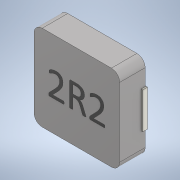
# Autodesk Inventor part: L_52x54x18mm
Saved by Autodesk Inventor 2020.3 (Build 243373000, 373)
## iProperties
Created: 2020-07-25
Part Number: L_52x54x18mm
Material: Generic
Document SubType Name: Modeling
Designer: franc
Density: 1 g/cm^3
Appearance: Default
Author: franc
Autodesk Inventor part; units mm, degrees
ref_plane "YZ Plane" through (0, 0, 0) normal (1, 0, 0) x (0, 1, 0)
ref_plane "XZ Plane" through (0, 0, 0) normal (0, 1, 0) x (-1, 0, 0)
ref_plane "XY Plane" through (0, 0, 0) normal (0, 0, 1) x (1, 0, 0)
sketch "Sketch1" plane through (0, 0, 0) normal (0, 0, 1) x (1, 0, 0)
  line L0 (-2.6, 2.6) -> (2.6, 2.6)
  line L1 (2.6, 2.6) -> (2.6, -2.6)
  line L2 (2.6, -2.6) -> (-2.6, -2.6)
  line L3 (-2.6, -2.6) -> (-2.6, 2.6)
  line L4 (-2.6, 2.6) -> (2.6, -2.6) construction
  line L5 (2.6, 2.6) -> (-2.6, -2.6) construction
  point P0 (0, 0)
  dimension "d0" = 5.2
  dimension "d1" = 5.2
  constraints: 12 end point, 2 midpoint, 2 parallel, 1 horizontal, 1 perpendicular
  measures "d0" distance of L0.start L0.end
  measures "d1" distance of L0.end L1.end
extrude "Extrusion1" add sketch "Sketch1" along normal blind 1.55
sketch "Sketch2" plane through (0, 0, 0) normal (0, 0, -1) x (-1, 0, 0)
  line L0 (-1.5, -1.1) -> (-2.7, -1.1)
  line L1 (-2.7, -1.1) -> (-2.7, 1.1)
  line L2 (-2.7, 1.1) -> (-1.5, 1.1)
  line L3 (-1.5, 1.1) -> (-1.5, -1.1)
  line L4 (-1.5, -1.1) -> (-2.7, 1.1) construction
  line L5 (-2.7, -1.1) -> (-1.5, 1.1) construction
  line L6 (-2.6, -2.6) -> (-2.6, 2.6) construction
  line L7 (-2.6, 0) -> (2.6, 0) construction
  line L8 (2.6, 2.6) -> (2.6, -2.6) construction
  line L9 (-2.6, 2.6) -> (2.6, 2.6) construction
  line L10 (0, 2.6) -> (0, 0) construction
  line L11 (1.5, -1.1) -> (2.7, -1.1)
  line L12 (2.7, -1.1) -> (2.7, 1.1)
  line L13 (2.7, 1.1) -> (1.5, 1.1)
  line L14 (1.5, 1.1) -> (1.5, -1.1)
  point P0 (-2.1, 0)
  point P1 (-2.1, 0)
  point P2 (2.1, 0)
  point P3 (2.1, 0)
  dimension "d4" = 1.2
  dimension "d5" = 0.1
  dimension "d6" = 2.2
  dimension "d7" = 5.4
  constraints: 24 end point, 6 midpoint, 6 symmetric about line, 2 parallel, 1 horizontal, 1 perpendicular, 1 point on line, 1 vertical
  measures "d4" distance of L0.start L0.end
  measures "d5" distance between parallel lines of L6 L1
  measures "d6" distance of L0.end L1.end
  measures "d7" distance between parallel lines of L12 L1
extrude "Extrusion2" add sketch "Sketch2" along normal blind 0.05 and the other way blind 0.25
fillet "Fillet1" radius 0.5 4 edges at (2.6, 2.6, 0.775) (-2.6, 2.6, 0.775) (2.6, -2.6, 0.775) (-2.6, -2.6, 0.775)
sketch "Sketch3" plane through (0, 0, 1.55) normal (0, 0, 1) x (1, 0, 0)
  line L0 (-2.5, 1.25) -> (2.5, 1.25) construction
  line L1 (2.5, 1.25) -> (2.5, -1.25) construction
  line L2 (2.5, -1.25) -> (-2.5, -1.25) construction
  line L3 (-2.5, -1.25) -> (-2.5, 1.25) construction
  line L4 (2.1, 2.6) -> (-2.1, 2.6) construction
  line L5 (0, 2.6) -> (0, -2.6) construction
  line L6 (-2.1, -2.6) -> (2.1, -2.6) construction
  line L7 (-2.6, 1.1) -> (-2.6, -1.1) construction
  line L8 (-2.6, 0) -> (2.6, 0) construction
  line L9 (2.6, -1.1) -> (2.6, 1.1) construction
  spline S0 degree 2 poles (-0.7725, -0.6683) (-0.7725, -0.6894) (-0.7782, -0.7218) (-0.788, -0.7444) (-0.8063, -0.7542) (-0.8162, -0.7542) knots 0 0 0 1 2 3 4 4 4
  line L10 (-0.8162, -0.7542) -> (-1.6415, -0.7542)
  spline S1 degree 2 poles (-1.6415, -0.7542) (-1.6585, -0.7542) (-1.6824, -0.7458) (-1.6993, -0.7275) (-1.7077, -0.6923) (-1.7077, -0.6669) knots 0 0 0 1 2 3 4 4 4
  spline S2 degree 2 poles (-1.7077, -0.6669) (-1.7077, -0.6444) (-1.7035, -0.6092) (-1.6923, -0.5824) (-1.6739, -0.557) (-1.6599, -0.5415) knots 0 0 0 1 2 3 4 4 4
  line L11 (-1.6599, -0.5415) -> (-1.3613, -0.2345)
  spline S3 degree 2 poles (-1.3613, -0.2345) (-1.257, -0.1289) (-1.1317, 0.0401) (-1.0641, 0.1782) (-1.043, 0.2908) (-1.043, 0.3415) knots 0 0 0 1 2 3 4 4 4
  spline S4 degree 2 poles (-1.043, 0.3415) (-1.043, 0.3908) (-1.0768, 0.4796) (-1.1401, 0.5458) (-1.2345, 0.5852) (-1.2965, 0.5852) knots 0 0 0 1 2 3 4 4 4
  spline S5 degree 2 poles (-1.2965, 0.5852) (-1.3697, 0.5852) (-1.4852, 0.5458) (-1.5725, 0.5007) (-1.6303, 0.4613) (-1.6444, 0.4613) knots 0 0 0 1 2 3 4 4 4
  spline S6 degree 2 poles (-1.6444, 0.4613) (-1.6528, 0.4613) (-1.6669, 0.4711) (-1.6754, 0.4908) (-1.6796, 0.5261) (-1.6796, 0.55) knots 0 0 0 1 2 3 4 4 4
  spline S7 degree 2 poles (-1.6796, 0.55) (-1.6796, 0.5669) (-1.6768, 0.5923) (-1.6711, 0.612) (-1.6627, 0.6275) (-1.6345, 0.6514) (-1.5669, 0.6937) (-1.4641, 0.7331) (-1.3401, 0.7613) (-1.2725, 0.7613) knots 0 0 0 1 2 3 4 5 6 7 8 8 8
  spline S8 degree 2 poles (-1.2725, 0.7613) (-1.1641, 0.7613) (-1.0007, 0.7007) (-0.8937, 0.5937) (-0.8401, 0.4528) (-0.8401, 0.3739) knots 0 0 0 1 2 3 4 4 4
  spline S9 degree 2 poles (-0.8401, 0.3739) (-0.8401, 0.3021) (-0.8655, 0.1599) (-0.9472, -0.0049) (-1.1021, -0.2063) (-1.2317, -0.3387) knots 0 0 0 1 2 3 4 4 4
  line L12 (-1.2317, -0.3387) -> (-1.4683, -0.5852)
  line L13 (-1.4683, -0.5852) -> (-0.8176, -0.5852)
  spline S10 degree 2 poles (-0.8176, -0.5852) (-0.8077, -0.5852) (-0.7908, -0.5951) (-0.7782, -0.6162) (-0.7725, -0.6472) (-0.7725, -0.6683) knots 0 0 0 1 2 3 4 4 4
  spline S11 degree 2 poles (0.5528, -0.7246) (0.5528, -0.7331) (0.5458, -0.7472) (0.5232, -0.757) (0.481, -0.7613) (0.4472, -0.7613) knots 0 0 0 1 2 3 4 4 4
  spline S12 degree 2 poles (0.4472, -0.7613) (0.4162, -0.7613) (0.3782, -0.757) (0.3556, -0.7458) (0.343, -0.7275) (0.3387, -0.7134) knots 0 0 0 1 2 3 4 4 4
  line L14 (0.3387, -0.7134) -> (0.2007, -0.3627)
  spline S13 degree 2 poles (0.2007, -0.3627) (0.1768, -0.3021) (0.1246, -0.2021) (0.0528, -0.1303) (-0.043, -0.0894) (-0.112, -0.0894) knots 0 0 0 1 2 3 4 4 4
  line L15 (-0.112, -0.0894) -> (-0.2444, -0.0894)
  line L16 (-0.2444, -0.0894) -> (-0.2444, -0.7246)
  spline S14 degree 2 poles (-0.2444, -0.7246) (-0.2444, -0.7331) (-0.2542, -0.7472) (-0.2768, -0.7556) (-0.3148, -0.7613) (-0.343, -0.7613) knots 0 0 0 1 2 3 4 4 4
  spline S15 degree 2 poles (-0.343, -0.7613) (-0.3725, -0.7613) (-0.4106, -0.7556) (-0.4331, -0.7472) (-0.443, -0.7331) (-0.443, -0.7246) knots 0 0 0 1 2 3 4 4 4
  line L17 (-0.443, -0.7246) -> (-0.443, 0.6585)
  spline S16 degree 2 poles (-0.443, 0.6585) (-0.443, 0.7035) (-0.3951, 0.7387) (-0.3697, 0.7387) knots 0 0 0 1 2 2 2
  line L18 (-0.3697, 0.7387) -> (-0.0514, 0.7387)
  spline S17 degree 2 poles (-0.0514, 0.7387) (0.0049, 0.7387) (0.0796, 0.7331) (0.1092, 0.7289) knots 0 0 0 1 2 2 2
  spline S18 degree 2 poles (0.1092, 0.7289) (0.1965, 0.7148) (0.3289, 0.65) (0.419, 0.55) (0.4641, 0.4218) (0.4641, 0.3444) knots 0 0 0 1 2 3 4 4 4
  spline S19 degree 2 poles (0.4641, 0.3444) (0.4641, 0.2697) (0.4232, 0.1514) (0.3472, 0.0599) (0.2415, -0.0077) (0.1754, -0.0303) knots 0 0 0 1 2 3 4 4 4
  spline S20 degree 2 poles (0.1754, -0.0303) (0.212, -0.0472) (0.2725, -0.0965) (0.3246, -0.1655) (0.3711, -0.2556) (0.3937, -0.312) knots 0 0 0 1 2 3 4 4 4
  line L19 (0.3937, -0.312) -> (0.5275, -0.6401)
  spline S21 degree 2 poles (0.5275, -0.6401) (0.5444, -0.6824) (0.5528, -0.7148) (0.5528, -0.7246) knots 0 0 0 1 2 2 2
  spline S22 degree 2 poles (0.2542, 0.3246) (0.2542, 0.412) (0.1754, 0.5331) (0.0838, 0.5599) knots 0 0 0 1 2 2 2
  spline S23 degree 2 poles (0.0838, 0.5599) (0.0542, 0.5683) (-0.0176, 0.5754) (-0.0768, 0.5754) knots 0 0 0 1 2 2 2
  line L20 (-0.0768, 0.5754) -> (-0.2444, 0.5754)
  line L21 (-0.2444, 0.5754) -> (-0.2444, 0.0711)
  line L22 (-0.2444, 0.0711) -> (-0.05, 0.0711)
  spline S24 degree 2 poles (-0.05, 0.0711) (0.0275, 0.0711) (0.143, 0.1092) (0.219, 0.1782) (0.2542, 0.2697) (0.2542, 0.3246) knots 0 0 0 1 2 3 4 4 4
  spline S25 degree 2 poles (1.7077, -0.6683) (1.7077, -0.6894) (1.7021, -0.7218) (1.6923, -0.7444) (1.6739, -0.7542) (1.6641, -0.7542) knots 0 0 0 1 2 3 4 4 4
  line L23 (1.6641, -0.7542) -> (0.8387, -0.7542)
  spline S26 degree 2 poles (0.8387, -0.7542) (0.8218, -0.7542) (0.7979, -0.7458) (0.781, -0.7275) (0.7725, -0.6923) (0.7725, -0.6669) knots 0 0 0 1 2 3 4 4 4
  spline S27 degree 2 poles (0.7725, -0.6669) (0.7725, -0.6444) (0.7768, -0.6092) (0.788, -0.5824) (0.8063, -0.557) (0.8204, -0.5415) knots 0 0 0 1 2 3 4 4 4
  line L24 (0.8204, -0.5415) -> (1.119, -0.2345)
  spline S28 degree 2 poles (1.119, -0.2345) (1.2232, -0.1289) (1.3486, 0.0401) (1.4162, 0.1782) (1.4373, 0.2908) (1.4373, 0.3415) knots 0 0 0 1 2 3 4 4 4
  spline S29 degree 2 poles (1.4373, 0.3415) (1.4373, 0.3908) (1.4035, 0.4796) (1.3401, 0.5458) (1.2458, 0.5852) (1.1838, 0.5852) knots 0 0 0 1 2 3 4 4 4
  spline S30 degree 2 poles (1.1838, 0.5852) (1.1106, 0.5852) (0.9951, 0.5458) (0.9077, 0.5007) (0.85, 0.4613) (0.8359, 0.4613) knots 0 0 0 1 2 3 4 4 4
  spline S31 degree 2 poles (0.8359, 0.4613) (0.8275, 0.4613) (0.8134, 0.4711) (0.8049, 0.4908) (0.8007, 0.5261) (0.8007, 0.55) knots 0 0 0 1 2 3 4 4 4
  spline S32 degree 2 poles (0.8007, 0.55) (0.8007, 0.5669) (0.8035, 0.5923) (0.8092, 0.612) (0.8176, 0.6275) (0.8458, 0.6514) (0.9134, 0.6937) (1.0162, 0.7331) (1.1401, 0.7613) (1.2077, 0.7613) knots 0 0 0 1 2 3 4 5 6 7 8 8 8
  spline S33 degree 2 poles (1.2077, 0.7613) (1.3162, 0.7613) (1.4796, 0.7007) (1.5866, 0.5937) (1.6401, 0.4528) (1.6401, 0.3739) knots 0 0 0 1 2 3 4 4 4
  spline S34 degree 2 poles (1.6401, 0.3739) (1.6401, 0.3021) (1.6148, 0.1599) (1.5331, -0.0049) (1.3782, -0.2063) (1.2486, -0.3387) knots 0 0 0 1 2 3 4 4 4
  line L25 (1.2486, -0.3387) -> (1.012, -0.5852)
  line L26 (1.012, -0.5852) -> (1.6627, -0.5852)
  spline S35 degree 2 poles (1.6627, -0.5852) (1.6725, -0.5852) (1.6894, -0.5951) (1.7021, -0.6162) (1.7077, -0.6472) (1.7077, -0.6683) knots 0 0 0 1 2 3 4 4 4
  point P0 (0, 0)
  dimension "d13" = 5
  dimension "d14" = 2.5
  constraints: 4 end point, 4 midpoint, 1 symmetric about line, 3 other
  measures "d13" distance of L2.end L1.end
  measures "d14" distance of L1.end L0.end
extrude "Extrusion4" cut sketch "Sketch3" against normal blind 0.01
body "Solid1"
